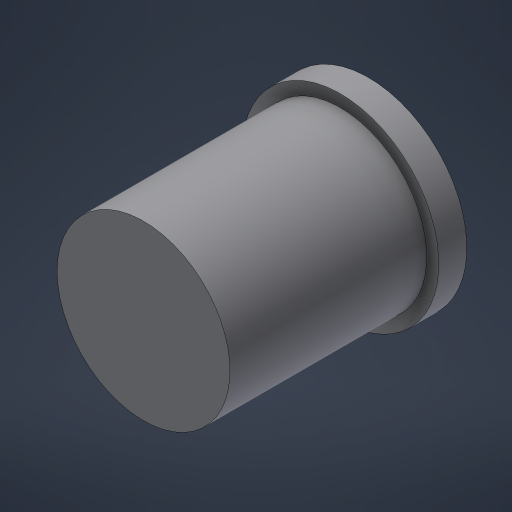
# Autodesk Inventor part: sw1
Saved by Autodesk Inventor 2023.5 (Build 275446000, 446)
## iProperties
Created: 2025-04-14
Part Number: sw1
Material: Generisch
Document SubType Name: Modeling
Designer: David Lill
Density: 1 g/cm^3
Appearance: Vorgabe
Author: David Lill
Autodesk Inventor part; units mm, degrees
ref_plane "YZ Plane" through (0, 0, 0) normal (1, 0, 0) x (0, 1, 0)
ref_plane "XZ Plane" through (0, 0, 0) normal (0, 1, 0) x (-1, 0, 0)
ref_plane "XY Plane" through (0, 0, 0) normal (0, 0, 1) x (1, 0, 0)
sketch "Skizze1" plane through (0, 0, 0) normal (0, 0, 1) x (1, 0, 0)
  line L0 (0, 0) -> (-6.15, 0)
  line L1 (-6.15, 0) -> (-6.15, 14)
  line L2 (-6.15, 14) -> (-7, 14)
  line L3 (-7, 14) -> (-7, 16)
  line L4 (-7, 16) -> (0, 16)
  line L5 (0, 16) -> (0, 0)
  dimension "d0" = 12.3
  dimension "d1" = 14
  dimension "d2" = 14
  dimension "d3" = 2
  constraints: 12 end point, 5 perpendicular, 1 horizontal
  measures "d0" diameter of L1 L5
  measures "d1" distance of L0.end L1.end
  measures "d2" diameter of L3 L5
  measures "d3" distance of L2.end L3.end
revolve "Umdrehung1" add sketch "Skizze1" angle 360 about axis through (0, 16, 0) along (0, -1, 0)
